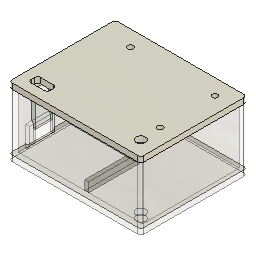
CO2SensorCase v1.3 (Autodesk Fusion 360 design; units mm, degrees)
Autodesk Fusion 360 part; units mm, degrees
sketch "BaseSketch" plane through (0, 0, 0) normal (0, 0, 1) x (1, 0, 0)
  line L0 (-35, 26.5) -> (0, 26.5)
  line L1 (0, 26.5) -> (0, 0)
  line L2 (0, 0) -> (-35, 0)
  line L3 (-35, 0) -> (-35, 26.5)
  line L4 (-30, 47.95) -> (27.5, 47.95)
  line L5 (27.5, 47.95) -> (27.5, 13.25)
  line L6 (27.5, 13.25) -> (-30, 13.25)
  line L7 (-30, 13.25) -> (-30, 47.95)
  circle A0 centre (-20.5, 44.65) radius 1.5
  circle A1 centre (24, 44.65) radius 1.5
  circle A2 centre (24, 15.65) radius 1.5
  line L8 (24, 44.65) -> (24, 15.65) construction
  line L9 (-20.5, 44.65) -> (24, 44.65) construction
  line L10 (-35, 13.25) -> (-37, 13.25) construction
  line L11 (-37, 13.25) -> (-37, 17.75)
  line L12 (-37, 17.75) -> (-35, 17.75)
  line L13 (-35, 13.25) -> (0, 13.25)
  line L14 (-37, 13.25) -> (-37, 8.75)
  line L15 (-37, 8.75) -> (-35, 8.75)
  line L16 (-37, 52.95) -> (32.5, 52.95)
  line L17 (32.5, 52.95) -> (32.5, -3)
  line L18 (32.5, -3) -> (-37, -3)
  line L19 (-37, -3) -> (-37, 52.95)
  line L20 (-30, 28.5) -> (0, 28.5)
  line L21 (0, 28.5) -> (0, 26.5)
  line L22 (0, 26.5) -> (-30, 26.5)
  line L23 (-30, 26.5) -> (-30, 28.5)
  line L24 (0, 28.5) -> (2, 28.5)
  line L25 (2, 28.5) -> (2, 13.25)
  line L26 (2, 13.25) -> (0, 13.25)
  line L27 (0, 13.25) -> (0, 28.5)
  line L28 (-0.5197, 0) -> (27.5, 0)
  line L29 (27.5, 0) -> (27.5, 13.25)
  line L30 (27.5, 13.25) -> (-0.5197, 13.25)
  line L31 (-0.5197, 13.25) -> (-0.5197, 0)
  line L32 (-35, 26.5) -> (-30, 26.5)
  line L33 (-30, 26.5) -> (-30, 47.95)
  line L34 (-30, 47.95) -> (-35, 47.95)
  line L35 (-35, 47.95) -> (-35, 26.5)
  line L36 (-35, 47.95) -> (27.5, 47.95)
  line L37 (27.5, 47.95) -> (27.5, 50.95)
  line L38 (27.5, 50.95) -> (-35, 50.95)
  line L39 (-35, 50.95) -> (-35, 47.95)
  line L40 (27.5, 50.95) -> (30.5, 50.95)
  line L41 (30.5, 50.95) -> (30.5, 0)
  line L42 (30.5, 0) -> (27.5, 0)
  line L43 (27.5, 0) -> (27.5, 50.95)
  line L44 (2, 13.25) -> (0, 13.25)
  line L45 (0, 13.25) -> (0, 0)
  line L46 (0, 0) -> (2, 0)
  line L47 (2, 0) -> (2, 13.25)
  line L48 (-30, 28.5) -> (-35, 28.5)
  line L49 (-35, 28.5) -> (-35, 26.5)
  line L50 (-35, 26.5) -> (-30, 26.5)
  line L51 (-30, 26.5) -> (-30, 28.5)
  dimension "d1" = 26.5
  dimension "d2" = 35
  dimension "d5" = 57.5
  dimension "d6" = 34.7
  dimension "d7" = 3
  dimension "d9" = 9.5
  dimension "d10" = 3
  dimension "d11" = 44.5
  dimension "d12" = 3
  dimension "d13" = 29
  dimension "d14" = 2.4
  dimension "d16" = 2
  dimension "d17" = 4.5
  dimension "d18" = 5
  dimension "d19" = 3
  dimension "d20" = 5
  dimension "d21" = 5
  dimension "d39" = 2
  dimension "d40" = 2
  dimension "d60" = 2
  dimension "d61" = 2
  constraint horizontal L0
  constraint vertical L1
  constraint horizontal L2
  constraint vertical L3
  constraint horizontal L4
  constraint vertical L5
  constraint horizontal L6
  constraint vertical L7
  constraint coincident A1.centre L8.start
  constraint coincident A2.centre L8.end
  constraint vertical L8
  constraint coincident A0.centre L9.start
  constraint horizontal L9
  constraint coincident L1.end L2.start
  constraint midpoint L3 L10.start
  constraint perpendicular L3 L10
  constraint perpendicular L10 L11
  constraint coincident L3 L12.end
  constraint perpendicular L3 L12
  constraint midpoint L1 L13.end
  constraint symmetric L11.start L10 L14.start
  constraint symmetric L10 L11.end L14.end
  constraint symmetric L10 L12.end L15.end
  constraint collinear L6 L13
  constraint horizontal L16
  constraint vertical L17
  constraint horizontal L18
  constraint vertical L19
  constraint collinear L11 L19
  constraint horizontal L20
  constraint vertical L21
  constraint horizontal L22
  constraint vertical L23
  constraint coincident L7 L20.start
  constraint horizontal L24
  constraint vertical L25
  constraint horizontal L26
  constraint vertical L27
  constraint coincident L6 L25.end
  constraint horizontal L28
  constraint vertical L29
  constraint horizontal L30
  constraint vertical L31
  constraint coincident L2 L28.start
  constraint horizontal L32
  constraint vertical L33
  constraint horizontal L34
  constraint vertical L35
  constraint horizontal L36
  constraint vertical L37
  constraint horizontal L38
  constraint vertical L39
  constraint collinear L5 L37
  constraint horizontal L40
  constraint vertical L41
  constraint horizontal L42
  constraint vertical L43
  constraint horizontal L44
  constraint vertical L45
  constraint horizontal L46
  constraint vertical L47
  constraint horizontal L48
  constraint vertical L49
  constraint horizontal L50
  constraint vertical L51
  measures "d1" distance of L0 L2
  measures "d2" distance of L1 L3
  measures "d5" distance of L4.start L4.end
  measures "d6" distance of L4.end L5.end
  measures "d7" diameter of A0
  measures "d9" distance of L7 A0.centre
  measures "d10" diameter of A1
  measures "d11" distance of A0.centre A1.centre
  measures "d12" diameter of A2
  measures "d13" vertical distance of A1.centre A2.centre
  measures "d14" distance of L6 A2.centre
  measures "d16" distance of L10.start L10.end
  measures "d17" distance of L10.end L11.end
  measures "d18" distance of L3 L7
  measures "d19" distance of L2 L18
  measures "d20" distance of L4 L16
  measures "d21" distance of L5 L17
  measures "d39" distance of L25 L27
  measures "d40" distance of L20 L22
  measures "d60" distance of L16 L38
  measures "d61" distance of L17 L41
extrude "MainBody" add sketch "BaseSketch" against normal blind 30 contours L2 L3 L12 L15 L16 L17 L18 L19 L28 L35 L38 L39 L40 L41 L42 L46 L49 makes body 1
extrude "Extrude2" add sketch "BaseSketch" along normal blind 3 separate body makes body 2
sketch "BottomInset" plane through (0, 0, -30) normal (0, 0, -1) x (1, 0, 0)
  line L0 (-35, -17.75) -> (-37, -17.75)
  line L1 (-37, -17.75) -> (-37, -52.95)
  line L2 (-37, -52.95) -> (32.5, -52.95)
  line L3 (32.5, -52.95) -> (32.5, 3)
  line L4 (32.5, 3) -> (-37, 3)
  line L5 (-37, 3) -> (-37, -8.75)
  line L6 (-37, -8.75) -> (-35, -8.75)
  line L7 (-35, -8.75) -> (-35, 0)
  line L8 (-35, 0) -> (30.5, 0)
  line L9 (-35, -50.95) -> (-35, -17.75)
  line L10 (32.5, 3) -> (-37, 3)
  line L11 (32.5, -52.95) -> (32.5, 3)
  line L12 (-37, -52.95) -> (32.5, -52.95)
  line L13 (-37, 3) -> (-37, -52.95)
  line L14 (30.5, -50.95) -> (-35, -50.95)
  line L15 (30.5, 0) -> (30.5, -50.95)
extrude "Extrude3" add sketch "BottomInset" along normal blind 3 separate body makes body 3
extrude "USBPortTopper" add sketch "BaseSketch" against normal blind 24 separate body contours L3 L11 L12 L14 L15 L19 makes body 4
sketch "Sketch3" plane through (0, 0, 3) normal (0, 0, 1) x (-1, 0, 0)
  circle A0 centre (-24, -44.65) radius 1.5
  circle A1 centre (20.5, -44.65) radius 1.5
  circle A2 centre (-24, -15.65) radius 1.5
  line L0 (37, 3) -> (-32.5, 3)
  line L1 (-32.5, 3) -> (-32.5, -52.95)
  line L2 (-32.5, -52.95) -> (37, -52.95)
  line L3 (37, -52.95) -> (37, 3)
  line L4 (0, 0) -> (35, 0)
  line L5 (35, 0) -> (35, -26.5)
  line L6 (-32.5, 3) -> (37, 3)
  line L7 (37, 3) -> (37, -52.95)
  line L8 (30.5, -2) -> (23.5, -2)
  line L9 (22, -3.5) -> (22, -5.5)
  line L10 (23.5, -7) -> (30.5, -7)
  line L11 (32, -5.5) -> (32, -3.5)
  circle A3 centre (-24.5, -5) radius 2.5
  line L12 (-32.5, -52.95) -> (-32.5, 3)
  arc A4 (30.5, -7) -> (32, -5.5) centre (30.5, -5.5) ccw
  arc A5 (32, -3.5) -> (30.5, -2) centre (30.5, -3.5) ccw
  arc A6 (23.5, -2) -> (22, -3.5) centre (23.5, -3.5) ccw
  arc A7 (22, -5.5) -> (23.5, -7) centre (23.5, -5.5) ccw
  line L13 (37, -52.95) -> (-32.5, -52.95)
  line L14 (-30.5, -50.95) -> (-30.5, 0)
  line L15 (-27.5, -50.95) -> (-30.5, -50.95)
  line L16 (-27.5, -50.95) -> (35, -50.95)
  line L17 (35, -47.95) -> (35, -26.5)
  line L18 (35, -50.95) -> (35, -47.95)
  line L19 (35, -50.95) -> (35, -17.75)
  line L20 (35, 0) -> (-30.5, 0)
  line L21 (35, -8.75) -> (35, 0)
  line L22 (35, -17.75) -> (35, 0)
  line L23 (0, -1) -> (34, -1)
  line L24 (34, -17.75) -> (34, -1)
  line L25 (34, -49.95) -> (34, -17.75)
  line L26 (-27.5, -49.95) -> (34, -49.95)
  line L27 (-27.5, -49.95) -> (-29.5, -49.95)
  line L28 (-29.5, -49.95) -> (-29.5, 0)
  line L29 (-30.5, 0) -> (0, 0)
  line L30 (-29.5, -49.95) -> (-29.5, -1)
  line L31 (-29.5, -1) -> (0, -1)
  line L32 (0, -1) -> (34, -1)
  line L33 (34, -17.75) -> (34, -1)
  line L34 (34, -49.95) -> (34, -17.75)
  line L35 (-27.5, -49.95) -> (34, -49.95)
  line L36 (-27.5, -49.95) -> (-29.5, -49.95)
  line L37 (35, -17.75) -> (35, -8.75)
  line L38 (32, -3) -> (32, -26.5)
  line L39 (32, -47.95) -> (32, -26.5)
  line L40 (-27.5, -47.95) -> (32, -47.95)
  line L41 (-27.5, -47.95) -> (-27.5, -3)
  line L42 (-27.5, -3) -> (0, -3)
  line L43 (0, -3) -> (32, -3)
  point P0 (32, -2)
  point P1 (22, -2)
  point P2 (32, -7)
  point P3 (35, -13.25)
  dimension "d30" = 10
  dimension "d31" = 5
  dimension "d32" = 5
  dimension "d33" = 5
  dimension "d35" = 5
  dimension "d36" = 8
  dimension "d37" = 8
  dimension "d43" = 1.5
  dimension "d44" = 1.5
  dimension "d45" = 1.5
  dimension "d68" = 1
  dimension "d69" = 1
  dimension "d70" = 3
  constraint horizontal L8
  constraint vertical L9
  constraint horizontal L10
  constraint vertical L11
  constraint coincident P2 L10
  constraint coincident P2 L11
  constraint tangent L10 A4
  constraint tangent L11 A4
  constraint coincident P0 L8
  constraint coincident P0 L11
  constraint tangent L8 A5
  constraint tangent L11 A5
  constraint coincident P1 L8
  constraint coincident P1 L9
  constraint tangent L8 A6
  constraint tangent L9 A6
  constraint equal A5 A6
  constraint tangent L9 A7
  constraint tangent L10 A7
  constraint coincident L19.end L22.start
  constraint coincident L4.end L5.start
  constraint coincident L14.end L20.end
  constraint coincident L4.start L29.end
  constraint coincident L21.start L37.end
  measures "d30" distance of P0 P1
  measures "d31" distance of P0 P2
  measures "d32" distance of L6 L8
  measures "d33" distance of L7 L11
  measures "d35" diameter of A3
  measures "d36" distance of A3.centre L12
  measures "d37" distance of L6 A3.centre
  measures "d43" radius of A4
  measures "d44" radius of A5
  measures "d45" radius of A7
extrude "Extrude8" add sketch "Sketch3" against normal blind 2 separate body contours L23 L24 L25 L26 L27 L28 L30 L31 L32 L33 L34 L35 L36 makes body 5
extrude "CutCaseHoles" cut sketch "Sketch3" against normal through all contours A3 L42 | A3 L42 bodies 3 2
extrude "Extrude5" cut sketch "Sketch3" against normal through all contours L8 A5 A6 L43 | L9 L10 L11 A4 A5 A6 A7 L38 L43 bodies 2
copy_body "CutPasteBodies1" bodies 2 removing the originals makes body 6 in component "TopLid"
copy_body "CutPasteBodies1'" bodies 1 3 4 removing the originals makes body 7 makes body 8 makes body 9 in component "BottomCase"
extrude "WemosBorderWall" add sketch "BaseSketch" along normal up to near side of body 8 separate body contours L0 L7 L23 L32 L33 L35 L48 L49 L50 L51 | L0 L7 L20 L21 L22 L23 L27 L33 L51 | L1 L6 L21 L24 L25 L26 L27 L30 L44 | L1 L6 L26 L28 L30 L44 L45 L46 L47 makes body 10
copy_body "CutPasteBodies2" bodies 10 removing the originals makes body 11 in component "BottomCase"
fillet "Fillet1" radius 1.5 4 edges at (32.5, -3, 1.5) (32.5, 52.95, 1.5) (-37, 52.95, 1.5) (-37, -3, 1.5) on bodies 6 in component "TopLid"
fillet "Fillet1'" radius 1.5 8 edges at (32.5, -3, -15) (32.5, 52.95, -15) (-37, 52.95, -15) (-37, -3, -15) (32.5, -3, -31.5) (32.5, 52.95, -31.5) (-37, 52.95, -31.5) (-37, -3, -31.5) on bodies 7 8 in component "BottomCase"
sketch "USBPortRecess" plane through (-37, 0, 0) normal (-1, 0, 0) x (0, -1, 0)
  line L0 (-51.45, 0) -> (-51.45, -30)
  line L1 (-51.45, -30) -> (-17.75, -30)
  line L2 (-17.75, -30) -> (-17.75, 0)
  line L3 (-17.75, 0) -> (-51.45, 0)
  line L4 (-17.75, 0) -> (-17.75, -30)
  line L5 (-8.75, -24) -> (-17.75, -24)
  line L6 (-8.75, 0) -> (-8.75, -30)
  line L7 (3, -30) -> (-52.95, -30)
  line L8 (-20.75, -21) -> (-5.75, -21)
  line L9 (-5.75, -21) -> (-5.75, -32)
  line L10 (-5.75, -32) -> (-20.75, -32)
  line L11 (-20.75, -32) -> (-20.75, -21)
  line L12 (-17.75, -29) -> (-8.75, -29)
  dimension "d51" = 3
  dimension "d52" = 3
  dimension "d53" = 2
  dimension "d55" = 3
  dimension "d77" = 5
  dimension "d81" = 1
  dimension "d82" = 5
  constraint horizontal L8
  constraint vertical L9
  constraint horizontal L10
  constraint vertical L11
  constraint coincident L4 L12.start
  constraint coincident L6 L12.end
  constraint perpendicular L6 L12
  measures "d51" distance of L6 L9
  measures "d52" distance of L4 L11
  measures "d53" distance of L7 L10
  measures "d55" distance of L5 L8
  measures "d81" distance of L7 L12
  measures "d82" distance of L5 L12
extrude "USBPortInset" cut sketch "USBPortRecess" against normal blind 1 contours L1 L2 L4 L7 L8 L11 | L1 L7 L9 L10 L11 | L2 L4 L5 L6 L8 | L6 L7 L8 L9 bodies 7 8 9 in component "BottomCase"
fillet "Fillet2" radius 1 8 edges at (-36, 20.75, -25.5) (-36, 19.25, -21) (-36, 7.25, -21) (-36, 5.75, -25.5) (-36, 13.25, -32) (-36, 5.75, -31) (-36, 20.75, -31) (-36, 13.25, -21) on bodies 7 8 9 in component "BottomCase"
move_body "Move1" bodies 5 to x (1, 0, 0) y (0, 1, 0) z (0, 0, 1) at (0, 0, -3)
copy_body "CutPasteBodies2'" bodies 5 removing the originals makes body 12 in component "TopLid"
extrude "WemosWall" cut sketch "BaseSketch" against normal blind 25 contours L0 L7 L23 L32 L33 L35 L48 L49 L50 L51 | L0 L7 L20 L21 L22 L23 L27 L33 L51 | L1 L6 L21 L24 L25 L26 L27 L30 L44 | L1 L6 L26 L28 L30 L44 L45 L46 L47 bodies 11 in component "BottomCase"
component "TopLid" placed x (1, 0, 0) y (0, 1, 0) z (0, 0, 1) at (0, 0, 0)
component "BottomCase" placed x (1, 0, 0) y (0, 1, 0) z (0, 0, 1) at (0, 0, 0)
equation "d1 = WemosD1Width"
equation "d2 = WemosD1Length"
equation "d22 = -MainBodyHeight"
equation "d28 = -USBBlockerHeight"
equation "WemosD1Width = 26.5 mm"
equation "WemosD1Length = 35 mm"
equation "d74 = -( MainBodyHeight - 5 mm )"
equation "MainBodyHeight = 30 mm"
equation "USBPortHeight = 5 mm"
equation "USBBlockerHeight = MainBodyHeight - ( USBPortHeight + USBUnderPortHeight )"
equation "USBUnderPortHeight = 1 mm"
equation "d81 = USBUnderPortHeight"
named bodies: "MainBody", "TopLid", "BottomPlate", "USBPortFiller", "WemosBorderWall", "TopLid InnerLip"
